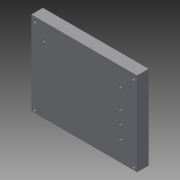
# Autodesk Inventor part: Board_Inventor_Part
Saved by Autodesk Inventor 2015 (Build 190159000, 159)
## iProperties
Created: 2016-10-04
Part Number: Board_Inventor_Part
Material: Generic
Document SubType Name: Modeling
Designer: stran
Density: 1 g/cm^3
Appearance: Default
Author: stran
Autodesk Inventor part; units mm, degrees
ref_plane "YZ Plane" through (0, 0, 0) normal (1, 0, 0) x (0, 1, 0)
ref_plane "XZ Plane" through (0, 0, 0) normal (0, 1, 0) x (-1, 0, 0)
ref_plane "XY Plane" through (0, 0, 0) normal (0, 0, 1) x (1, 0, 0)
sketch "Sketch1" plane through (0, 0, 0) normal (0, 0, 1) x (1, 0, 0)
  line L0 (0, 0) -> (116.51, 0)
  line L1 (116.51, 0) -> (116.51, 92.2428)
  line L2 (116.51, 92.2428) -> (0, 92.2428)
  line L3 (0, 92.2428) -> (0, 0)
  dimension "d0" = 92.2428
  dimension "d1" = 116.51
  constraints: 8 end point, 2 parallel, 1 horizontal, 1 perpendicular
  measures "d0" distance of L2.end L0.start
  measures "d1" distance of L0.start L0.end
extrude "Extrusion1" add sketch "Sketch1" along normal blind 12.7
sketch "Sketch2" plane through (0, 0, 12.7) normal (0, 0, 1) x (1, 0, 0)
  line L0 (0, 92.2428) -> (0, 0) projected
  line L1 (0, 0) -> (116.51, 0) projected
  point P0 (3.683, 87.1982)
  point P1 (3.2004, 3.048)
  point P2 (112.5474, 3.2258)
  point P3 (112.3696, 87.1474)
  dimension "d4" = 3.2004
  dimension "d5" = 3.048
  dimension "d6" = 112.5474
  dimension "d7" = 3.2258
  dimension "d8" = 3.683
  dimension "d9" = 87.1982
  dimension "d10" = 112.3696
  dimension "d11" = 87.1474
  measures "d4" distance from line of L0 point (3.2, 3.048)
  measures "d5" distance from line of L1 point (3.2, 3.048)
  measures "d6" distance from line of L0 point (112.547, 3.226)
  measures "d7" distance from line of L1 point (112.547, 3.226)
  measures "d8" distance from line of L0 point (3.683, 87.198)
  measures "d9" distance from line of point (3.683, 87.198) L1
  measures "d10" distance from line of point (112.37, 87.147) L0
  measures "d11" distance from line of L1 point (112.37, 87.147)
hole "Hole1" at (3.683, 87.1982, 12.7) at (3.2004, 3.048, 12.7) at (112.5474, 3.2258, 12.7) at (112.3696, 87.1474, 12.7) direction (0, 0, -1) diameter 3.175 end through all
sketch "Sketch3" plane through (0, 0, 12.7) normal (0, 0, 1) x (1, 0, 0)
  line L0 (0, 92.2428) -> (0, 0) projected
  line L1 (0, 0) -> (116.51, 0) projected
  point P0 (13.97, 73.914)
  point P1 (97.79, 72.39)
  point P2 (97.79, 50.8)
  point P3 (97.79, 36.83)
  point P4 (97.79, 22.86)
  dimension "d19" = 13.97
  dimension "d20" = 73.914
  dimension "d21" = 97.79
  dimension "d22" = 72.39
  dimension "d23" = 97.79
  dimension "d24" = 97.79
  dimension "d25" = 97.79
  dimension "d26" = 50.8
  dimension "d27" = 36.83
  dimension "d28" = 22.86
  measures "d19" distance from line of L0 point (13.97, 73.914)
  measures "d20" distance from line of L1 point (13.97, 73.914)
  measures "d21" distance from line of L0 point (97.79, 72.39)
  measures "d22" distance from line of L1 point (97.79, 72.39)
  measures "d23" distance from line of L0 point (97.79, 50.8)
  measures "d24" distance from line of L0 point (97.79, 36.83)
  measures "d25" distance from line of L0 point (97.79, 22.86)
  measures "d26" distance from line of L1 point (97.79, 50.8)
  measures "d27" distance from line of L1 point (97.79, 36.83)
  measures "d28" distance from line of L1 point (97.79, 22.86)
hole "Hole2" at (13.97, 73.914, 12.7) at (97.79, 72.39, 12.7) at (97.79, 50.8, 12.7) at (97.79, 36.83, 12.7) at (97.79, 22.86, 12.7) direction (0, 0, -1) diameter 3.175 depth 0.254 tip angle 118
equation "\"d23\" = d21"
equation "\"d24\" = d23"
equation "\"d25\" = d24"
body "Solid1"
